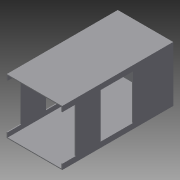
# Autodesk Inventor part: Cover
Saved by Autodesk Inventor 2015 SP1 (Build 190203100, 203)
## iProperties
Created: 2015-03-04
Part Number: Cover
Material: Generic
Document SubType Name: Modeling
Designer: Andrew
Density: 1 g/cm^3
Appearance: Default
Author: Andrew
Autodesk Inventor part; units mm, degrees
ref_plane "YZ Plane" through (0, 0, 0) normal (1, 0, 0) x (0, 1, 0)
ref_plane "XZ Plane" through (0, 0, 0) normal (0, 1, 0) x (-1, 0, 0)
ref_plane "XY Plane" through (0, 0, 0) normal (0, 0, 1) x (1, 0, 0)
sketch "Sketch1" plane through (0, 0, 0) normal (0, 1, 0) x (-1, 0, 0)
  line L0 (-100, 100) -> (100, 100)
  line L1 (100, 100) -> (100, -100)
  line L2 (100, -100) -> (-100, -100)
  line L3 (-100, -100) -> (-100, 100)
  line L4 (-100, 100) -> (100, -100) construction
  line L5 (100, 100) -> (-100, -100) construction
  line L6 (103.175, -103.175) -> (103.175, 103.175)
  line L7 (103.175, 103.175) -> (-103.175, 103.175)
  line L8 (-103.175, 103.175) -> (-103.175, -103.175)
  line L9 (-103.175, -103.175) -> (103.175, -103.175)
  point P0 (0, 0)
  dimension "d0" = 200
  dimension "d1" = 3.175
  constraints: 20 end point, 4 parallel, 3 perpendicular, 2 midpoint, 1 horizontal, 3 other
  measures "d0" distance between parallel lines of L3 L1
  measures "d1" distance between parallel lines of L1 L6
extrude "Extrusion1" add sketch "Sketch1" along normal blind 410
sketch "Sketch2" plane through (0, 410, 0) normal (0, 1, 0) x (1, 0, 0)
  line L0 (-100, -100) -> (-100, 100) projected
  line L1 (-100, 100) -> (100, 100) projected
  line L2 (100, 100) -> (100, -100) projected
  line L3 (100, -100) -> (-100, -100) projected
  line L4 (-103.175, 103.175) -> (-103.175, -103.175) projected
  line L5 (-103.175, -103.175) -> (103.175, -103.175) projected
  line L6 (103.175, -103.175) -> (103.175, 103.175) projected
  line L7 (103.175, 103.175) -> (-103.175, 103.175) projected
  point P0 (0, 0)
extrude "Extrusion2" add sketch "Sketch2" along normal blind 3.175 contours L0 L1 L2 L3 | L7 L6 L5 L4
sketch "Sketch3" plane through (103.175, 0, 103.175) normal (1, 0, 0) x (0, 0, -1)
  line L0 (0, 0) -> (206.35, 0) projected
  line L1 (206.35, 0) -> (206.35, 413.175) projected
  line L2 (0, 413.175) -> (206.35, 413.175) projected
  line L3 (0, 0) -> (0, 413.175) projected
  line L4 (206.35, 0) -> (0, 0) projected
  line L5 (186.35, 0) -> (186.35, 50)
  line L6 (186.35, 50) -> (20, 50)
  line L7 (20, 50) -> (20, 0)
  line L8 (20, 263.175) -> (20, 143.175)
  line L9 (20, 143.175) -> (186.35, 143.175)
  line L10 (186.35, 143.175) -> (186.35, 263.175)
  line L11 (186.35, 263.175) -> (20, 263.175)
  point P0 (103.175, 0)
  dimension "d6" = 50
  dimension "d7" = 20
  dimension "d8" = 20
  dimension "d9" = 150
  dimension "d12" = 120
  constraints: 14 end point, 4 perpendicular, 3 vertical, 2 collinear, 2 point on line
  measures "d6" distance of L6.end L7.end
  measures "d7" distance between parallel lines of L3 L7
  measures "d8" distance between parallel lines of L1 L5
  measures "d9" distance between parallel lines of L2 L11
  measures "d12" distance between parallel lines of L9 L11
extrude "Extrusion3" cut sketch "Sketch3" against normal up to surface (206.35 mm away) contours L7 L6 L5 L0 | L11 L10 L9 L8
body "Solid1"
